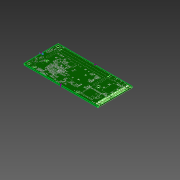
# Autodesk Inventor part: hw_LM - PCB
Saved by Autodesk Inventor 2018 (Build 220112000, 112)
## iProperties
Created: 2025-09-15
Part Number: hw_LM - PCB
Material: PCB
Document SubType Name: Modeling
Designer: mbs18
Density: 4 g/cm^3
Appearance: PCB
Mass: 49.92 g
Surface Area: 162.464 cm^2
Volume: 12.48 cm^3
Author: mbs18
Autodesk Inventor part; units mm, degrees
ref_plane "YZ Plane" through (0, 0, 0) normal (1, 0, 0) x (0, 1, 0)
ref_plane "XZ Plane" through (0, 0, 0) normal (0, 1, 0) x (-1, 0, 0)
ref_plane "XY Plane" through (0, 0, 0) normal (0, 0, 1) x (1, 0, 0)
sketch "Sketch1" plane through (0, 0, 0) normal (0, 0, 1) x (1, 0, 0)
  line L0 (54.6842, -25.25) -> (-54.6842, -25.25)
  line L1 (-54.6842, -25.25) -> (-54.6842, 25.25)
  line L2 (-54.6842, 25.25) -> (54.6842, 25.25)
  line L3 (54.6842, 25.25) -> (54.6842, -25.25)
  line L4 (54.6842, -25.25) -> (-54.6842, 25.25) construction
  line L5 (-54.6842, -25.25) -> (54.6842, 25.25) construction
  point P0 (0, 0)
  dimension "d0" = 109.3684
  dimension "d1" = 50.5
  constraints: 12 end point, 2 midpoint, 2 parallel, 1 horizontal, 1 perpendicular
  measures "d0" distance of L1.end L2.end
  measures "d1" distance of L0.end L1.end
extrude "Extrusion1" add sketch "Sketch1" against normal blind 1.6
ref_plane "Work Plane1" through (-54.6842, 0, 0) normal (0, 1, 0) x (1, 0, 0)
sketch "TOP 17122025" plane through (0, 0, 0) normal (0, 0, 1) x (1, 0, 0)
  line L0 (-54.6842, 25.25) -> (54.6842, 25.25) projected
  line L1 (-54.6842, -25.25) -> (-54.6842, 25.25) projected
  line L2 (54.6842, -25.25) -> (-54.6842, -25.25) projected
  line L3 (-54.6842, 25.2836) -> (54.6842, 25.2836) construction
  line L4 (54.6842, 25.2836) -> (54.6842, -25.2836) construction
  line L5 (54.6842, -25.2836) -> (-54.6842, -25.2836) construction
  line L6 (-54.6842, -25.2836) -> (-54.6842, 25.2836) construction
  point P0 (0, 25.25)
  point P1 (0, 25.2876)
  point P2 (0, 25.25)
  point P3 (-52.2223, 0)
  point P4 (-54.6842, 0)
  point P5 (0, 25.2836)
  point P6 (0, 25.25)
  point P7 (-55.0358, 0)
  point P8 (-54.6842, 0)
  point P9 (-54.7176, 0)
  point P10 (-54.6842, 0)
  point P11 (0, 25.2836)
  point P12 (0, 25.25)
  point P13 (0, 25.2836)
  point P14 (0, -25.25)
  point P15 (-54.7176, 0)
  point P16 (-54.6842, 0)
  point P17 (0, 25.2836)
  point P18 (-54.6842, 0)
  dimension "d295" = 109.3684
  constraints: 11 midpoint, 5 horizontal alignment, 5 vertical alignment, 2 other
  measures "d295" distance of L3.start L3.end
ref_plane "Work Plane3" through (0, 0, -1.6) normal (0, 0, 1) x (1, 0, 0)
sketch "BOTTOM 17122025" plane through (0, 0, -1.6) normal (0, 0, 1) x (1, 0, 0)
  line L0 (-54.6842, 25.25) -> (54.6842, 25.25) projected
  line L1 (-54.6842, -25.25) -> (-54.6842, 25.25) projected
  line L2 (54.6842, -25.25) -> (-54.6842, -25.25) projected
  line L3 (-54.6842, 25.2836) -> (54.6842, 25.2836) construction
  line L4 (54.6842, 25.2836) -> (54.6842, -25.2836) construction
  line L5 (54.6842, -25.2836) -> (-54.6842, -25.2836) construction
  line L6 (-54.6842, -25.2836) -> (-54.6842, 25.2836) construction
  point P0 (0, 25.2876)
  point P1 (0, 25.25)
  point P2 (-52.2223, 0)
  point P3 (-54.6842, 0)
  point P4 (0, 25.2836)
  point P5 (0, 25.25)
  point P6 (-52.22, 0)
  point P7 (-54.6842, 0)
  point P8 (0, 25.2836)
  point P9 (0, 25.25)
  point P10 (-54.7176, 0)
  point P11 (-54.6842, 0)
  point P12 (0, 25.2836)
  point P13 (0, -25.25)
  point P14 (-55.0334, 0)
  point P15 (-54.6842, 0)
  point P16 (0, 25.2836)
  point P17 (0, 25.25)
  point P18 (-54.6842, 0)
  point P19 (-54.6842, 0)
  dimension "d304" = 109.3684
  constraints: 12 midpoint, 5 vertical alignment, 4 horizontal alignment, 1 coincident, 2 other
  measures "d304" distance of L3.start L3.end
fillet "Fillet1" radius 0.8 4 edges at (54.6842, 25.25, -0.8) (54.6842, -25.25, -0.8) (-54.6842, -25.25, -0.8) (-54.6842, 25.25, -0.8)
ref_plane "Work Plane2" through (0, 0, -1.6) normal (0, 0, 1) x (1, 0, 0)
sketch "Sketch6" plane through (0, 0, 0) normal (0, 0, 1) x (1, 0, 0)
  line L0 (54.6842, 24.45) -> (54.6842, -24.45) projected
  line L1 (-53.8842, 25.25) -> (53.8842, 25.25) projected
  line L2 (53.8842, -25.25) -> (-53.8842, -25.25) projected
  point P0 (0, 0)
  point P1 (21.4842, -22)
  point P2 (-42.1158, -22)
  dimension "d54" = 33.2
  dimension "d56" = 63.6
  dimension "d76" = 3.25
  constraints: 1 horizontal alignment
  measures "d54" distance from line of L0 point (21.484, -22)
  measures "d56" distance of point (21.484, -22) point (-42.116, -22)
  measures "d76" distance from line of L2 point (21.484, -22)
hole "Hole2" at (21.4842, -22, 0) at (-42.1158, -22, 0) direction (0, 0, -1) diameter 3 end through all
sketch "Sketch7" plane through (0, 0, 0) normal (0, 0, 1) x (1, 0, 0)
  line L0 (54.6842, 24.45) -> (54.6842, -24.45) projected
  line L1 (54.6842, 20) -> (24.0842, 20) construction
  line L2 (54.6842, 20) -> (85.2842, 20) construction
  line L3 (53.8842, -25.25) -> (-53.8842, -25.25) projected
  line L4 (24.0842, 20) -> (-44.7158, 20) construction
  line L5 (-53.8842, 25.25) -> (53.8842, 25.25) projected
  point P0 (0, 0)
  dimension "d64" = 30.6
  dimension "d65" = 180
  dimension "d67" = 68.8
  dimension "d253" = 45.25
  constraints: 6 end point, 2 coincident, 2 collinear, 1 horizontal, 1 perpendicular, 1 point on line
  measures "d64" distance of L1.start L1.end
  measures "d65" angle of L1 L2
  measures "d67" distance of L4.start L4.end
  measures "d253" distance from line of L3 L4.start
hole "Hole3" at (24.0842, 20, 0) at (-44.7158, 20, 0) direction (0, 0, -1) diameter 1.65 end through all
sketch "Sketch12" plane through (0, 0, 0) normal (0, 0, 1) x (1, 0, 0)
  line L0 (-53.8842, 25.25) -> (53.8842, 25.25) projected
  line L1 (54.6842, 24.45) -> (54.6842, -24.45) projected
  point P0 (0, 0)
  point P1 (24.3092, 22)
  dimension "d105" = 3.25
  dimension "d106" = 30.375
  measures "d105" distance from line of L0 point (24.309, 22)
  measures "d106" distance from line of L1 point (24.309, 22)
hole "Hole4" at (24.3092, 22, 0) direction (0, 0, -1) diameter 0.7 depth 8 tip angle 118
sketch "Sketch14" plane through (0, 0, -1.6) normal (0, 0, -1) x (-1, 0, 0)
  point P0 (0, 0)
  point P1 (41.887, -3.6561)
  point P2 (40.6059, -3.6561)
  point P3 (41.887, -4.9219)
  point P4 (41.887, -6.1787)
  point P5 (41.887, -7.4622)
  point P6 (40.6059, -4.9219)
  point P7 (40.6059, -6.1787)
  point P8 (40.6059, -7.4622)
hole "Hole5" at (-41.887, -3.6561, -1.6) at (-40.6059, -3.6561, -1.6) at (-41.887, -4.9219, -1.6) at (-41.887, -6.1787, -1.6) at (-41.887, -7.4622, -1.6) at (-40.6059, -4.9219, -1.6) at (-40.6059, -6.1787, -1.6) at (-40.6059, -7.4622, -1.6) direction (0, 0, 1) diameter 0.5 end through all
sketch "Sketch15" plane through (0, 0, 0) normal (0, 0, 1) x (1, 0, 0)
  arc A0 (-54.6842, -24.45) -> (-53.8842, -25.25) centre (-53.8842, -24.45) ccw projected
  line L0 (-54.6842, -24.45) -> (-54.6842, 24.45) projected
  line L1 (53.8842, -25.25) -> (-53.8842, -25.25) projected
  circle A1 centre (-50.6842, -21.25) radius 3
  circle A2 centre (29.9842, 0) radius 3.7
  circle A3 centre (29.9842, 0) radius 3
  line L2 (54.6842, 24.45) -> (54.6842, -24.45) projected
  circle A4 centre (-50.6842, 21.25) radius 3
  line L3 (-53.8842, 25.25) -> (53.8842, 25.25) projected
  point P0 (0, 0)
  dimension "d238" = 6
  dimension "d239" = 7.4
  dimension "d240" = 6
  dimension "d254" = 24.7
  dimension "d255" = 4
  dimension "d256" = 4
  dimension "d257" = 6
  dimension "d258" = 4
  dimension "d259" = 4
  constraints: 4 centre point, 2 coincident
  measures "d238" diameter of A1
  measures "d239" diameter of A2
  measures "d240" diameter of A3
  measures "d254" distance from line of L2 A3.centre
  measures "d255" distance from line of A1.centre L0
  measures "d256" distance from line of L1 A1.centre
  measures "d257" diameter of A4
  measures "d258" distance from line of L3 A4.centre
  measures "d259" distance from line of A4.centre L0
hole "Hole6" at (-50.6842, 21.25, 0) at (-50.6842, -21.25, 0) at (29.9842, 0, 0) at (29.9842, 0, 0) at (29.9842, 0, 0) direction (0, 0, -1) diameter 3 end through all
sketch "Sketch16" plane through (0, 0, 0) normal (0, 0, 1) x (1, 0, 0)
  line L0 (54.1842, -23) -> (49.1842, -23)
  line L1 (49.1842, -23) -> (49.1842, -22)
  line L2 (49.1842, -22) -> (54.1842, -22)
  line L3 (54.1842, -22) -> (54.1842, -23)
  line L4 (54.1842, -23) -> (49.1842, -22) construction
  line L5 (49.1842, -23) -> (54.1842, -22) construction
  line L6 (53.8842, -25.25) -> (-53.8842, -25.25) projected
  line L7 (54.6842, 24.45) -> (54.6842, -24.45) projected
  line L8 (54.1842, -19.8) -> (49.1842, -19.8)
  line L9 (49.1842, -19.8) -> (49.1842, -19)
  line L10 (49.1842, -19) -> (54.1842, -19)
  line L11 (54.1842, -19) -> (54.1842, -19.8)
  line L12 (54.1842, -19.8) -> (49.1842, -19) construction
  line L13 (49.1842, -19.8) -> (54.1842, -19) construction
  line L14 (54.1842, -18.4) -> (49.1842, -18.4)
  line L15 (49.1842, -18.4) -> (49.1842, -17.6)
  line L16 (49.1842, -17.6) -> (54.1842, -17.6)
  line L17 (54.1842, -17.6) -> (54.1842, -18.4)
  line L18 (54.1842, -18.4) -> (49.1842, -17.6) construction
  line L19 (49.1842, -18.4) -> (54.1842, -17.6) construction
  line L20 (49.1842, -17) -> (54.1842, -17)
  line L21 (54.1842, -17) -> (54.1842, -16.2)
  line L22 (54.1842, -16.2) -> (49.1842, -16.2)
  line L23 (49.1842, -16.2) -> (49.1842, -17)
  line L24 (49.1842, -17) -> (54.1842, -16.2) construction
  line L25 (54.1842, -17) -> (49.1842, -16.2) construction
  line L26 (54.1842, -14.5) -> (49.1842, -14.5)
  line L27 (49.1842, -14.5) -> (49.1842, -15.3)
  line L28 (49.1842, -15.3) -> (54.1842, -15.3)
  line L29 (54.1842, -15.3) -> (54.1842, -14.5)
  line L30 (54.1842, -14.5) -> (49.1842, -15.3) construction
  line L31 (49.1842, -14.5) -> (54.1842, -15.3) construction
  line L32 (49.1842, -13.1) -> (54.1842, -13.1)
  line L33 (54.1842, -13.1) -> (54.1842, -13.9)
  line L34 (54.1842, -13.9) -> (49.1842, -13.9)
  line L35 (49.1842, -13.9) -> (49.1842, -13.1)
  line L36 (49.1842, -13.1) -> (54.1842, -13.9) construction
  line L37 (54.1842, -13.1) -> (49.1842, -13.9) construction
  line L38 (54.1842, -11.7) -> (49.1842, -11.7)
  line L39 (49.1842, -11.7) -> (49.1842, -12.5)
  line L40 (49.1842, -12.5) -> (54.1842, -12.5)
  line L41 (54.1842, -12.5) -> (54.1842, -11.7)
  line L42 (54.1842, -11.7) -> (49.1842, -12.5) construction
  line L43 (49.1842, -11.7) -> (54.1842, -12.5) construction
  line L44 (49.1842, -10) -> (54.1842, -10)
  line L45 (54.1842, -10) -> (54.1842, -10.8)
  line L46 (54.1842, -10.8) -> (49.1842, -10.8)
  line L47 (49.1842, -10.8) -> (49.1842, -10)
  line L48 (49.1842, -10) -> (54.1842, -10.8) construction
  line L49 (54.1842, -10) -> (49.1842, -10.8) construction
  line L50 (54.1842, -9.4) -> (49.1842, -9.4)
  line L51 (49.1842, -9.4) -> (49.1842, -8.6)
  line L52 (49.1842, -8.6) -> (54.1842, -8.6)
  line L53 (54.1842, -8.6) -> (54.1842, -9.4)
  line L54 (54.1842, -9.4) -> (49.1842, -8.6) construction
  line L55 (49.1842, -9.4) -> (54.1842, -8.6) construction
  line L56 (49.1842, -7.2) -> (54.1842, -7.2)
  line L57 (54.1842, -7.2) -> (54.1842, -8)
  line L58 (54.1842, -8) -> (49.1842, -8)
  line L59 (49.1842, -8) -> (49.1842, -7.2)
  line L60 (49.1842, -7.2) -> (54.1842, -8) construction
  line L61 (54.1842, -7.2) -> (49.1842, -8) construction
  line L62 (54.1842, -4) -> (49.1842, -4)
  line L63 (49.1842, -4) -> (49.1842, -5)
  line L64 (49.1842, -5) -> (54.1842, -5)
  line L65 (54.1842, -5) -> (54.1842, -4)
  line L66 (54.1842, -4) -> (49.1842, -5) construction
  line L67 (49.1842, -4) -> (54.1842, -5) construction
  line L68 (54.1842, -1.9) -> (49.1842, -1.9)
  line L69 (49.1842, -1.9) -> (49.1842, -1.1)
  line L70 (49.1842, -1.1) -> (54.1842, -1.1)
  line L71 (54.1842, -1.1) -> (54.1842, -1.9)
  line L72 (54.1842, -1.9) -> (49.1842, -1.1) construction
  line L73 (49.1842, -1.9) -> (54.1842, -1.1) construction
  line L74 (54.1842, 0.4) -> (49.1842, 0.4)
  line L75 (49.1842, 0.4) -> (49.1842, -0.4)
  line L76 (49.1842, -0.4) -> (54.1842, -0.4)
  line L77 (54.1842, -0.4) -> (54.1842, 0.4)
  line L78 (54.1842, 0.4) -> (49.1842, -0.4) construction
  line L79 (49.1842, 0.4) -> (54.1842, -0.4) construction
  line L80 (49.1842, 1.9) -> (54.1842, 1.9)
  line L81 (54.1842, 1.9) -> (54.1842, 1.1)
  line L82 (54.1842, 1.1) -> (49.1842, 1.1)
  line L83 (49.1842, 1.1) -> (49.1842, 1.9)
  line L84 (49.1842, 1.9) -> (54.1842, 1.1) construction
  line L85 (54.1842, 1.9) -> (49.1842, 1.1) construction
  line L86 (49.1842, 2.6) -> (54.1842, 2.6)
  line L87 (54.1842, 2.6) -> (54.1842, 3.4)
  line L88 (54.1842, 3.4) -> (49.1842, 3.4)
  line L89 (49.1842, 3.4) -> (49.1842, 2.6)
  line L90 (49.1842, 2.6) -> (54.1842, 3.4) construction
  line L91 (54.1842, 2.6) -> (49.1842, 3.4) construction
  line L92 (54.1842, 4.9) -> (49.1842, 4.9)
  line L93 (49.1842, 4.9) -> (49.1842, 4.1)
  line L94 (49.1842, 4.1) -> (54.1842, 4.1)
  line L95 (54.1842, 4.1) -> (54.1842, 4.9)
  line L96 (54.1842, 4.9) -> (49.1842, 4.1) construction
  line L97 (49.1842, 4.9) -> (54.1842, 4.1) construction
  line L98 (49.1842, 6.4) -> (54.1842, 6.4)
  line L99 (54.1842, 6.4) -> (54.1842, 5.6)
  line L100 (54.1842, 5.6) -> (49.1842, 5.6)
  line L101 (49.1842, 5.6) -> (49.1842, 6.4)
  line L102 (49.1842, 6.4) -> (54.1842, 5.6) construction
  line L103 (54.1842, 6.4) -> (49.1842, 5.6) construction
  line L104 (54.1842, 7.9) -> (49.1842, 7.9)
  line L105 (49.1842, 7.9) -> (49.1842, 7.1)
  line L106 (49.1842, 7.1) -> (54.1842, 7.1)
  line L107 (54.1842, 7.1) -> (54.1842, 7.9)
  line L108 (54.1842, 7.9) -> (49.1842, 7.1) construction
  line L109 (49.1842, 7.9) -> (54.1842, 7.1) construction
  line L110 (54.1842, 9.4) -> (49.1842, 9.4)
  line L111 (49.1842, 9.4) -> (49.1842, 8.6)
  line L112 (49.1842, 8.6) -> (54.1842, 8.6)
  line L113 (54.1842, 8.6) -> (54.1842, 9.4)
  line L114 (54.1842, 9.4) -> (49.1842, 8.6) construction
  line L115 (49.1842, 9.4) -> (54.1842, 8.6) construction
  line L116 (54.1842, 10.9) -> (49.1842, 10.9)
  line L117 (49.1842, 10.9) -> (49.1842, 10.1)
  line L118 (49.1842, 10.1) -> (54.1842, 10.1)
  line L119 (54.1842, 10.1) -> (54.1842, 10.9)
  line L120 (54.1842, 10.9) -> (49.1842, 10.1) construction
  line L121 (49.1842, 10.9) -> (54.1842, 10.1) construction
  line L122 (54.1842, 12.4) -> (49.1842, 12.4)
  line L123 (49.1842, 12.4) -> (49.1842, 11.6)
  line L124 (49.1842, 11.6) -> (54.1842, 11.6)
  line L125 (54.1842, 11.6) -> (54.1842, 12.4)
  line L126 (54.1842, 12.4) -> (49.1842, 11.6) construction
  line L127 (49.1842, 12.4) -> (54.1842, 11.6) construction
  line L128 (49.1842, 13.9) -> (54.1842, 13.9)
  line L129 (54.1842, 13.9) -> (54.1842, 13.1)
  line L130 (54.1842, 13.1) -> (49.1842, 13.1)
  line L131 (49.1842, 13.1) -> (49.1842, 13.9)
  line L132 (49.1842, 13.9) -> (54.1842, 13.1) construction
  line L133 (54.1842, 13.9) -> (49.1842, 13.1) construction
  line L134 (49.1842, 14.6) -> (54.1842, 14.6)
  line L135 (54.1842, 14.6) -> (54.1842, 15.4)
  line L136 (54.1842, 15.4) -> (49.1842, 15.4)
  line L137 (49.1842, 15.4) -> (49.1842, 14.6)
  line L138 (49.1842, 14.6) -> (54.1842, 15.4) construction
  line L139 (54.1842, 14.6) -> (49.1842, 15.4) construction
  line L140 (54.1842, 18.625) -> (49.1842, 18.625)
  line L141 (49.1842, 18.625) -> (49.1842, 17.375)
  line L142 (49.1842, 17.375) -> (54.1842, 17.375)
  line L143 (54.1842, 17.375) -> (54.1842, 18.625)
  line L144 (54.1842, 18.625) -> (49.1842, 17.375) construction
  line L145 (49.1842, 18.625) -> (54.1842, 17.375) construction
  line L146 (49.1842, 21.875) -> (54.1842, 21.875)
  line L147 (54.1842, 21.875) -> (54.1842, 23.125)
  line L148 (54.1842, 23.125) -> (49.1842, 23.125)
  line L149 (49.1842, 23.125) -> (49.1842, 21.875)
  line L150 (49.1842, 21.875) -> (54.1842, 23.125) construction
  line L151 (54.1842, 21.875) -> (49.1842, 23.125) construction
  point P0 (0, 0)
  point P1 (51.6842, -22.5)
  point P2 (51.6842, -19.4)
  point P3 (51.6842, -19.4)
  point P4 (51.6842, -22.5)
  point P5 (51.6842, -18)
  point P6 (51.6842, -16.6)
  point P7 (51.6842, -14.9)
  point P8 (51.6842, -13.5)
  point P9 (51.6842, -12.1)
  point P10 (51.6842, -12.1)
  point P11 (51.6842, -13.5)
  point P12 (51.6842, -14.9)
  point P13 (51.6842, -13.5)
  point P14 (51.6842, -16.6)
  point P15 (51.6842, -18)
  point P16 (51.6842, -16.6)
  point P17 (51.6842, -10.4)
  point P18 (51.6842, -9)
  point P19 (51.6842, -7.6)
  point P20 (51.6842, -7.6)
  point P21 (51.6842, -9)
  point P22 (51.6842, -10.4)
  point P23 (51.6842, -12.1)
  point P24 (51.6842, -10.4)
  point P25 (51.6842, -4.5)
  point P26 (51.6842, -4.5)
  point P27 (51.6842, -7.6)
  point P28 (51.6842, -1.5)
  point P29 (51.6842, -1.5)
  point P30 (51.6842, -4.5)
  point P31 (51.6842, 0)
  point P32 (51.6842, 0)
  point P33 (51.6842, -1.5)
  point P34 (51.6842, 1.5)
  point P35 (51.6842, 1.5)
  point P36 (51.6842, 0)
  point P37 (51.6842, 3)
  point P38 (51.6842, 4.5)
  point P39 (51.6842, 6)
  point P40 (51.6842, 7.5)
  point P41 (51.6842, 9)
  point P42 (51.6842, 10.5)
  point P43 (51.6842, 12)
  point P44 (51.6842, 13.5)
  point P45 (51.6842, 15)
  point P46 (51.6842, 18)
  point P47 (51.6842, 18)
  point P48 (51.6842, 15)
  point P49 (51.6842, 22.5)
  point P50 (51.6842, 22.5)
  point P51 (51.6842, 22.5)
  point P52 (51.6842, 18)
  dimension "d311" = 5
  dimension "d312" = 1
  dimension "d313" = 2.75
  dimension "d314" = 0.5
  dimension "d315" = 3.1
  dimension "d316" = 5
  dimension "d317" = 0.8
  dimension "d318" = 5
  dimension "d319" = 0.8
  dimension "d320" = 1.4
  dimension "d321" = 0.5
  dimension "d322" = 5
  dimension "d323" = 0.8
  dimension "d324" = 5
  dimension "d325" = 0.8
  dimension "d326" = 5
  dimension "d327" = 0.8
  dimension "d328" = 1.4
  dimension "d329" = 1.7
  dimension "d330" = 1.4
  dimension "d331" = 5
  dimension "d332" = 0.8
  dimension "d333" = 1.4
  dimension "d334" = 5
  dimension "d335" = 0.8
  dimension "d336" = 1.7
  dimension "d337" = 5
  dimension "d338" = 0.8
  dimension "d339" = 5
  dimension "d340" = 0.8
  dimension "d341" = 1.4
  dimension "d342" = 1.4
  dimension "d343" = 5
  dimension "d344" = 1
  dimension "d345" = 3.1
  dimension "d346" = 5
  dimension "d347" = 0.8
  dimension "d348" = 3
  dimension "d349" = 5
  dimension "d350" = 0.8
  dimension "d351" = 1.5
  dimension "d352" = 5
  dimension "d353" = 0.8
  dimension "d354" = 1.5
  dimension "d355" = 5
  dimension "d356" = 0.8
  dimension "d357" = 5
  dimension "d358" = 0.8
  dimension "d359" = 5
  dimension "d360" = 0.8
  dimension "d361" = 1.5
  dimension "d362" = 1.5
  dimension "d363" = 1.5
  dimension "d364" = 5
  dimension "d365" = 0.8
  dimension "d366" = 5
  dimension "d367" = 0.8
  dimension "d368" = 5
  dimension "d369" = 0.8
  dimension "d370" = 5
  dimension "d371" = 0.8
  dimension "d372" = 5
  dimension "d373" = 0.8
  dimension "d374" = 5
  constraints: 300 end point, 77 midpoint, 50 parallel, 25 horizontal, 25 perpendicular, 23 vertical alignment
  measures "d311" distance of L1.end L2.end
  measures "d312" distance of L0.end L1.end
  measures "d313" distance from line of L6 point (51.684, -22.5)
  measures "d314" distance between parallel lines of L7 L3
  measures "d315" distance of point (51.684, -22.5) point (51.684, -19.4)
  measures "d316" distance of L8.start L8.end
  measures "d317" distance of L8.end L9.end
  measures "d318" distance of L15.end L16.end
  measures "d319" distance of L14.end L15.end
  measures "d320" distance of point (51.684, -19.4) point (51.684, -18)
  measures "d321" distance between parallel lines of L7 L17
  measures "d322" distance of L22.end L21.end
  measures "d323" distance of L21.end L20.end
  measures "d324" distance of L28.end L27.end
  measures "d325" distance of L27.end L26.end
  measures "d326" distance of L33.end L34.end
  measures "d327" distance of L32.end L33.end
  measures "d328" distance of point (51.684, -18) point (51.684, -16.6)
  measures "d329" distance of point (51.684, -14.9) point (51.684, -16.6)
  measures "d330" distance of point (51.684, -13.5) point (51.684, -14.9)
  measures "d331" distance of L40.end L39.end
  measures "d332" distance of L39.end L38.end
  measures "d333" distance of point (51.684, -12.1) point (51.684, -13.5)
  measures "d334" distance of L45.end L46.end
  measures "d335" distance of L44.end L45.end
  measures "d336" distance of point (51.684, -12.1) point (51.684, -10.4)
  measures "d337" distance of L51.end L52.end
  measures "d338" distance of L50.end L51.end
  measures "d339" distance of L57.end L58.end
  measures "d340" distance of L56.end L57.end
  measures "d341" distance of point (51.684, -9) point (51.684, -10.4)
  measures "d342" distance of point (51.684, -9) point (51.684, -7.6)
  measures "d343" distance of L64.end L63.end
  measures "d344" distance of L63.end L62.end
  measures "d345" distance of point (51.684, -7.6) point (51.684, -4.5)
  measures "d346" distance of L69.end L70.end
  measures "d347" distance of L68.end L69.end
  measures "d348" distance of point (51.684, -4.5) point (51.684, -1.5)
  measures "d349" distance of L76.end L75.end
  measures "d350" distance of L75.end L74.end
  measures "d351" distance of point (51.684, -1.5) point (51.684, 0)
  measures "d352" distance of L81.end L82.end
  measures "d353" distance of L80.end L81.end
  measures "d354" distance of point (51.684, 0) point (51.684, 1.5)
  measures "d355" distance of L88.end L87.end
  measures "d356" distance of L87.end L86.end
  measures "d357" distance of L94.end L93.end
  measures "d358" distance of L93.end L92.end
  measures "d359" distance of L99.end L100.end
  measures "d360" distance of L98.end L99.end
  measures "d361" distance between parallel lines of L88 L80
  measures "d362" distance between parallel lines of L92 L88
  measures "d363" distance between parallel lines of L98 L92
  measures "d364" distance of L106.end L105.end
  measures "d365" distance of L105.end L104.end
  measures "d366" distance of L112.end L111.end
  measures "d367" distance of L111.end L110.end
  measures "d368" distance of L118.end L117.end
  measures "d369" distance of L117.end L116.end
  measures "d370" distance of L124.end L123.end
  measures "d371" distance of L123.end L122.end
  measures "d372" distance of L129.end L130.end
  measures "d373" distance of L128.end L129.end
  measures "d374" distance of L136.end L135.end
extrude "Extrusion2" add sketch "Sketch16" along normal blind 0.5
sketch "Sketch17" plane through (0, 0, -1.6) normal (0, 0, -1) x (-1, 0, 0)
  line L0 (-49.1842, -23.8) -> (-54.1842, -23.8)
  line L1 (-54.1842, -23.8) -> (-54.1842, -23)
  line L2 (-54.1842, -23) -> (-49.1842, -23)
  line L3 (-49.1842, -23) -> (-49.1842, -23.8)
  line L4 (-49.1842, -23.8) -> (-54.1842, -23) construction
  line L5 (-54.1842, -23.8) -> (-49.1842, -23) construction
  line L6 (-54.1842, -21.2) -> (-49.1842, -21.2)
  line L7 (-49.1842, -21.2) -> (-49.1842, -22)
  line L8 (-49.1842, -22) -> (-54.1842, -22)
  line L9 (-54.1842, -22) -> (-54.1842, -21.2)
  line L10 (-54.1842, -21.2) -> (-49.1842, -22) construction
  line L11 (-49.1842, -21.2) -> (-54.1842, -22) construction
  line L12 (-54.1842, -19.1) -> (-49.1842, -19.1)
  line L13 (-49.1842, -19.1) -> (-49.1842, -19.9)
  line L14 (-49.1842, -19.9) -> (-54.1842, -19.9)
  line L15 (-54.1842, -19.9) -> (-54.1842, -19.1)
  line L16 (-54.1842, -19.1) -> (-49.1842, -19.9) construction
  line L17 (-49.1842, -19.1) -> (-54.1842, -19.9) construction
  line L18 (-54.1842, -17.6) -> (-49.1842, -17.6)
  line L19 (-49.1842, -17.6) -> (-49.1842, -18.4)
  line L20 (-49.1842, -18.4) -> (-54.1842, -18.4)
  line L21 (-54.1842, -18.4) -> (-54.1842, -17.6)
  line L22 (-54.1842, -17.6) -> (-49.1842, -18.4) construction
  line L23 (-49.1842, -17.6) -> (-54.1842, -18.4) construction
  line L24 (-54.1842, -16.1) -> (-49.1842, -16.1)
  line L25 (-49.1842, -16.1) -> (-49.1842, -16.9)
  line L26 (-49.1842, -16.9) -> (-54.1842, -16.9)
  line L27 (-54.1842, -16.9) -> (-54.1842, -16.1)
  line L28 (-54.1842, -16.1) -> (-49.1842, -16.9) construction
  line L29 (-49.1842, -16.1) -> (-54.1842, -16.9) construction
  line L30 (-53.8842, -25.25) -> (53.8842, -25.25) projected
  line L31 (-54.6842, 24.45) -> (-54.6842, -24.45) projected
  line L32 (-49.1842, -14.8) -> (-54.1842, -14.8)
  line L33 (-54.1842, -14.8) -> (-54.1842, -14)
  line L34 (-54.1842, -14) -> (-49.1842, -14)
  line L35 (-49.1842, -14) -> (-49.1842, -14.8)
  line L36 (-49.1842, -14.8) -> (-54.1842, -14) construction
  line L37 (-54.1842, -14.8) -> (-49.1842, -14) construction
  line L38 (-54.1842, -12.2) -> (-49.1842, -12.2)
  line L39 (-49.1842, -12.2) -> (-49.1842, -13)
  line L40 (-49.1842, -13) -> (-54.1842, -13)
  line L41 (-54.1842, -13) -> (-54.1842, -12.2)
  line L42 (-54.1842, -12.2) -> (-49.1842, -13) construction
  line L43 (-49.1842, -12.2) -> (-54.1842, -13) construction
  line L44 (-54.1842, -10.1) -> (-49.1842, -10.1)
  line L45 (-49.1842, -10.1) -> (-49.1842, -10.9)
  line L46 (-49.1842, -10.9) -> (-54.1842, -10.9)
  line L47 (-54.1842, -10.9) -> (-54.1842, -10.1)
  line L48 (-54.1842, -10.1) -> (-49.1842, -10.9) construction
  line L49 (-49.1842, -10.1) -> (-54.1842, -10.9) construction
  line L50 (-49.1842, -9.4) -> (-54.1842, -9.4)
  line L51 (-54.1842, -9.4) -> (-54.1842, -8.6)
  line L52 (-54.1842, -8.6) -> (-49.1842, -8.6)
  line L53 (-49.1842, -8.6) -> (-49.1842, -9.4)
  line L54 (-49.1842, -9.4) -> (-54.1842, -8.6) construction
  line L55 (-54.1842, -9.4) -> (-49.1842, -8.6) construction
  line L56 (-54.1842, -7.1) -> (-49.1842, -7.1)
  line L57 (-49.1842, -7.1) -> (-49.1842, -7.9)
  line L58 (-49.1842, -7.9) -> (-54.1842, -7.9)
  line L59 (-54.1842, -7.9) -> (-54.1842, -7.1)
  line L60 (-54.1842, -7.1) -> (-49.1842, -7.9) construction
  line L61 (-49.1842, -7.1) -> (-54.1842, -7.9) construction
  line L62 (-54.1842, -1.1) -> (-49.1842, -1.1)
  line L63 (-49.1842, -1.1) -> (-49.1842, -1.9)
  line L64 (-49.1842, -1.9) -> (-54.1842, -1.9)
  line L65 (-54.1842, -1.9) -> (-54.1842, -1.1)
  line L66 (-54.1842, -1.1) -> (-49.1842, -1.9) construction
  line L67 (-49.1842, -1.1) -> (-54.1842, -1.9) construction
  line L68 (-54.1842, 0.4) -> (-49.1842, 0.4)
  line L69 (-49.1842, 0.4) -> (-49.1842, -0.4)
  line L70 (-49.1842, -0.4) -> (-54.1842, -0.4)
  line L71 (-54.1842, -0.4) -> (-54.1842, 0.4)
  line L72 (-54.1842, 0.4) -> (-49.1842, -0.4) construction
  line L73 (-49.1842, 0.4) -> (-54.1842, -0.4) construction
  line L74 (-54.1842, 1.9) -> (-49.1842, 1.9)
  line L75 (-49.1842, 1.9) -> (-49.1842, 1.1)
  line L76 (-49.1842, 1.1) -> (-54.1842, 1.1)
  line L77 (-54.1842, 1.1) -> (-54.1842, 1.9)
  line L78 (-54.1842, 1.9) -> (-49.1842, 1.1) construction
  line L79 (-49.1842, 1.9) -> (-54.1842, 1.1) construction
  line L80 (-54.1842, 3.4) -> (-49.1842, 3.4)
  line L81 (-49.1842, 3.4) -> (-49.1842, 2.6)
  line L82 (-49.1842, 2.6) -> (-54.1842, 2.6)
  line L83 (-54.1842, 2.6) -> (-54.1842, 3.4)
  line L84 (-54.1842, 3.4) -> (-49.1842, 2.6) construction
  line L85 (-49.1842, 3.4) -> (-54.1842, 2.6) construction
  line L86 (-49.1842, 4.9) -> (-54.1842, 4.9)
  line L87 (-54.1842, 4.9) -> (-54.1842, 4.1)
  line L88 (-54.1842, 4.1) -> (-49.1842, 4.1)
  line L89 (-49.1842, 4.1) -> (-49.1842, 4.9)
  line L90 (-49.1842, 4.9) -> (-54.1842, 4.1) construction
  line L91 (-54.1842, 4.9) -> (-49.1842, 4.1) construction
  line L92 (-54.1842, 6.4) -> (-49.1842, 6.4)
  line L93 (-49.1842, 6.4) -> (-49.1842, 5.6)
  line L94 (-49.1842, 5.6) -> (-54.1842, 5.6)
  line L95 (-54.1842, 5.6) -> (-54.1842, 6.4)
  line L96 (-54.1842, 6.4) -> (-49.1842, 5.6) construction
  line L97 (-49.1842, 6.4) -> (-54.1842, 5.6) construction
  line L98 (-49.1842, 7.1) -> (-54.1842, 7.1)
  line L99 (-54.1842, 7.1) -> (-54.1842, 7.9)
  line L100 (-54.1842, 7.9) -> (-49.1842, 7.9)
  line L101 (-49.1842, 7.9) -> (-49.1842, 7.1)
  line L102 (-49.1842, 7.1) -> (-54.1842, 7.9) construction
  line L103 (-54.1842, 7.1) -> (-49.1842, 7.9) construction
  line L104 (-54.1842, 9.4) -> (-49.1842, 9.4)
  line L105 (-49.1842, 9.4) -> (-49.1842, 8.6)
  line L106 (-49.1842, 8.6) -> (-54.1842, 8.6)
  line L107 (-54.1842, 8.6) -> (-54.1842, 9.4)
  line L108 (-54.1842, 9.4) -> (-49.1842, 8.6) construction
  line L109 (-49.1842, 9.4) -> (-54.1842, 8.6) construction
  line L110 (-54.1842, 10.9) -> (-49.1842, 10.9)
  line L111 (-49.1842, 10.9) -> (-49.1842, 10.1)
  line L112 (-49.1842, 10.1) -> (-54.1842, 10.1)
  line L113 (-54.1842, 10.1) -> (-54.1842, 10.9)
  line L114 (-54.1842, 10.9) -> (-49.1842, 10.1) construction
  line L115 (-49.1842, 10.9) -> (-54.1842, 10.1) construction
  line L116 (-54.1842, 12.4) -> (-49.1842, 12.4)
  line L117 (-49.1842, 12.4) -> (-49.1842, 11.6)
  line L118 (-49.1842, 11.6) -> (-54.1842, 11.6)
  line L119 (-54.1842, 11.6) -> (-54.1842, 12.4)
  line L120 (-54.1842, 12.4) -> (-49.1842, 11.6) construction
  line L121 (-49.1842, 12.4) -> (-54.1842, 11.6) construction
  line L122 (-54.1842, 13.9) -> (-49.1842, 13.9)
  line L123 (-49.1842, 13.9) -> (-49.1842, 13.1)
  line L124 (-49.1842, 13.1) -> (-54.1842, 13.1)
  line L125 (-54.1842, 13.1) -> (-54.1842, 13.9)
  line L126 (-54.1842, 13.9) -> (-49.1842, 13.1) construction
  line L127 (-49.1842, 13.9) -> (-54.1842, 13.1) construction
  line L128 (-54.1842, 15.4) -> (-49.1842, 15.4)
  line L129 (-49.1842, 15.4) -> (-49.1842, 14.6)
  line L130 (-49.1842, 14.6) -> (-54.1842, 14.6)
  line L131 (-54.1842, 14.6) -> (-54.1842, 15.4)
  line L132 (-54.1842, 15.4) -> (-49.1842, 14.6) construction
  line L133 (-49.1842, 15.4) -> (-54.1842, 14.6) construction
  line L134 (-54.1842, 18.625) -> (-49.1842, 18.625)
  line L135 (-49.1842, 18.625) -> (-49.1842, 17.375)
  line L136 (-49.1842, 17.375) -> (-54.1842, 17.375)
  line L137 (-54.1842, 17.375) -> (-54.1842, 18.625)
  line L138 (-54.1842, 18.625) -> (-49.1842, 17.375) construction
  line L139 (-49.1842, 18.625) -> (-54.1842, 17.375) construction
  line L140 (-54.1842, 23.125) -> (-49.1842, 23.125)
  line L141 (-49.1842, 23.125) -> (-49.1842, 21.875)
  line L142 (-49.1842, 21.875) -> (-54.1842, 21.875)
  line L143 (-54.1842, 21.875) -> (-54.1842, 23.125)
  line L144 (-54.1842, 23.125) -> (-49.1842, 21.875) construction
  line L145 (-49.1842, 23.125) -> (-54.1842, 21.875) construction
  point P0 (0, 0)
  point P1 (-51.6842, -23.4)
  point P2 (-51.6842, -21.6)
  point P3 (-51.6842, -19.5)
  point P4 (-51.6842, -18)
  point P5 (-51.6842, -16.5)
  point P6 (-51.6842, -14.4)
  point P7 (-51.6842, -12.6)
  point P8 (-51.6842, -10.5)
  point P9 (-51.6842, -9)
  point P10 (-51.6842, -7.5)
  point P11 (-51.6842, -1.5)
  point P12 (-51.6842, 0)
  point P13 (-51.6842, 1.5)
  point P14 (-51.6842, 3)
  point P15 (-51.6842, 4.5)
  point P16 (-51.6842, 6)
  point P17 (-51.6842, 7.5)
  point P18 (-51.6842, 9)
  point P19 (-51.6842, 10.5)
  point P20 (-51.6842, 12)
  point P21 (-51.6842, 13.5)
  point P22 (-51.6842, 15)
  point P23 (-51.6842, 18)
  point P24 (-51.6842, 22.5)
  dimension "d390" = 5
  dimension "d391" = 0.8
  dimension "d392" = 5
  dimension "d393" = 0.8
  dimension "d394" = 5
  dimension "d395" = 0.8
  dimension "d396" = 5
  dimension "d397" = 0.8
  dimension "d398" = 5
  dimension "d399" = 0.8
  dimension "d400" = 1.85
  dimension "d401" = 1.8
  dimension "d402" = 2.1
  dimension "d403" = 1.5
  dimension "d404" = 1.5
  dimension "d405" = 0.5
  dimension "d406" = 5
  dimension "d407" = 0.8
  dimension "d408" = 0.5
  dimension "d409" = 2.1
  dimension "d410" = 5
  dimension "d411" = 0.8
  dimension "d414" = 1.8
  dimension "d415" = 0.5
  dimension "d416" = 5
  dimension "d417" = 0.8
  dimension "d418" = 2.1
  dimension "d419" = 0.5
  dimension "d420" = 5
  dimension "d421" = 0.8
  dimension "d422" = 0.5
  dimension "d423" = 1.5
  dimension "d424" = 5
  dimension "d425" = 0.8
  dimension "d426" = 1.5
  dimension "d427" = 0.5
  dimension "d428" = 5
  dimension "d429" = 0.8
  dimension "d430" = 6
  dimension "d431" = 5
  dimension "d432" = 0.8
  dimension "d433" = 5
  dimension "d434" = 0.8
  dimension "d435" = 1.5
  dimension "d436" = 1.5
  dimension "d437" = 5
  dimension "d438" = 0.8
  dimension "d439" = 5
  dimension "d440" = 0.8
  dimension "d441" = 5
  dimension "d442" = 0.8
  dimension "d443" = 5
  dimension "d444" = 0.8
  dimension "d445" = 5
  dimension "d446" = 0.8
  dimension "d447" = 5
  dimension "d448" = 0.8
  dimension "d449" = 5
  dimension "d450" = 0.8
  dimension "d451" = 5
  dimension "d452" = 0.8
  dimension "d453" = 5
  dimension "d454" = 0.8
  dimension "d455" = 1.5
  constraints: 288 end point, 48 midpoint, 48 parallel, 24 horizontal, 24 perpendicular, 14 vertical alignment
  measures "d390" distance of L1.end L2.end
  measures "d391" distance of L0.end L1.end
  measures "d392" distance of L7.end L8.end
  measures "d393" distance of L6.end L7.end
  measures "d394" distance of L13.end L14.end
  measures "d395" distance of L12.end L13.end
  measures "d396" distance of L19.end L20.end
  measures "d397" distance of L18.end L19.end
  measures "d398" distance of L25.end L26.end
  measures "d399" distance of L24.end L25.end
  measures "d400" distance from line of L30 point (-51.684, -23.4)
  measures "d401" distance of point (-51.684, -23.4) point (-51.684, -21.6)
  measures "d402" distance of point (-51.684, -21.6) point (-51.684, -19.5)
  measures "d403" distance of point (-51.684, -19.5) point (-51.684, -18)
  measures "d404" distance of point (-51.684, -18) point (-51.684, -16.5)
  measures "d405" distance between parallel lines of L1 L31
  measures "d406" distance of L33.end L34.end
  measures "d407" distance of L32.end L33.end
  measures "d408" distance between parallel lines of L33 L31
  measures "d409" distance of point (-51.684, -16.5) point (-51.684, -14.4)
  measures "d410" distance of L39.end L40.end
  measures "d411" distance of L38.end L39.end
  measures "d414" distance between parallel lines of L32 L40
  measures "d415" distance between parallel lines of L31 L41
  measures "d416" distance of L45.end L46.end
  measures "d417" distance of L44.end L45.end
  measures "d418" distance of point (-51.684, -12.6) point (-51.684, -10.5)
  measures "d419" distance between parallel lines of L31 L47
  measures "d420" distance of L51.end L52.end
  measures "d421" distance of L50.end L51.end
  measures "d422" distance between parallel lines of L31 L51
  measures "d423" distance of point (-51.684, -10.5) point (-51.684, -9)
  measures "d424" distance of L57.end L58.end
  measures "d425" distance of L56.end L57.end
  measures "d426" distance of point (-51.684, -9) point (-51.684, -7.5)
  measures "d427" distance between parallel lines of L31 L59
  measures "d428" distance of L63.end L64.end
  measures "d429" distance of L62.end L63.end
  measures "d430" distance of point (-51.684, -1.5) point (-51.684, -7.5)
  measures "d431" distance of L69.end L70.end
  measures "d432" distance of L68.end L69.end
  measures "d433" distance of L75.end L76.end
  measures "d434" distance of L74.end L75.end
  measures "d435" distance of point (-51.684, 0) point (-51.684, -1.5)
  measures "d436" distance of point (-51.684, 0) point (-51.684, 1.5)
  measures "d437" distance of L81.end L82.end
  measures "d438" distance of L80.end L81.end
  measures "d439" distance of L88.end L87.end
  measures "d440" distance of L87.end L86.end
  measures "d441" distance of L93.end L94.end
  measures "d442" distance of L92.end L93.end
  measures "d443" distance of L99.end L100.end
  measures "d444" distance of L98.end L99.end
  measures "d445" distance of L105.end L106.end
  measures "d446" distance of L104.end L105.end
  measures "d447" distance of L111.end L112.end
  measures "d448" distance of L110.end L111.end
  measures "d449" distance of L117.end L118.end
  measures "d450" distance of L116.end L117.end
  measures "d451" distance of L123.end L124.end
  measures "d452" distance of L122.end L123.end
  measures "d453" distance of L129.end L130.end
  measures "d454" distance of L128.end L129.end
  measures "d455" distance of point (-51.684, 3) point (-51.684, 1.5)
extrude "Extrusion3" add sketch "Sketch17" along normal blind 0.5
body "Solid1"
